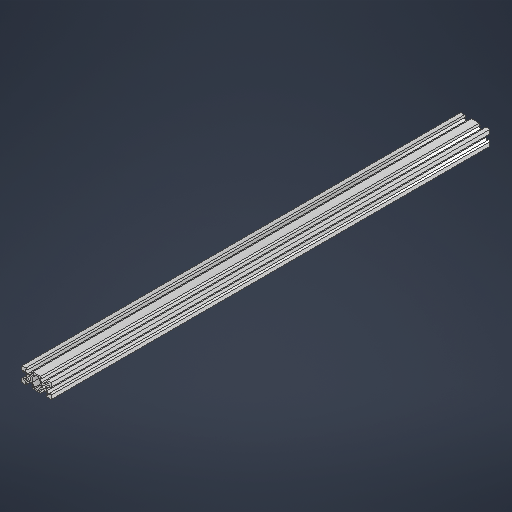
# Autodesk Inventor part: vslot_2040_100mm
Saved by Autodesk Inventor 2026 (Build 300175050, 175E)
## iProperties
Created: 2025-11-10
Part Number: vslot_2040_100mm
Material: Generic
Document SubType Name: Modeling
Designer: habbo
Density: 1 g/cm^3
Appearance: Aluminum - Polished
Author: habbo
Autodesk Inventor part; units mm, degrees
ref_plane "YZ Plane" through (0, 0, 0) normal (1, 0, 0) x (0, 1, 0)
ref_plane "XZ Plane" through (0, 0, 0) normal (0, 1, 0) x (-1, 0, 0)
ref_plane "XY Plane" through (0, 0, 0) normal (0, 0, 1) x (1, 0, 0)
sketch "Sketch1" plane through (0, 0, 0) normal (0, 0, 1) x (1, 0, 0)
  line L0 (4.5, 8.2) -> (4.5, 6.5562)
  line L1 (6.9, 8.2) -> (4.5, 8.2)
  line L2 (5.3896, 10) -> (6.9, 8.2)
  line L3 (-5.3896, 10) -> (5.3896, 10)
  line L4 (-5.3896, 10) -> (-6.9, 8.2)
  line L5 (-6.9, 8.2) -> (-4.5, 8.2)
  line L6 (-4.5, 8.2) -> (-4.5, 6.5562)
  line L7 (-4.5, 6.5562) -> (-7.1607, 3.9)
  line L8 (-9.4804, 3.8998) -> (-7.1607, 3.9)
  line L9 (-9.4804, 3.8998) -> (-10, 3.5998)
  line L10 (-10.5196, 3.8998) -> (-10, 3.5998)
  line L11 (-12.8393, 3.9) -> (-10.5196, 3.8998)
  line L12 (-15.5, 6.5562) -> (-12.8393, 3.9)
  line L13 (-15.5, 8.2) -> (-15.5, 6.5562)
  line L14 (-13.1, 8.2) -> (-15.5, 8.2)
  line L15 (-14.6104, 10) -> (-13.1, 8.2)
  line L16 (-20, 10) -> (-14.6104, 10)
  line L17 (-20, 10) -> (-20, 4.6104)
  line L18 (-20, 4.6104) -> (-18.2, 3.1)
  line L19 (-18.2, 3.1) -> (-18.2, 5.5)
  line L20 (-16.5562, 5.5) -> (-18.2, 5.5)
  line L21 (-16.5562, 5.5) -> (-13.9, 2.8393)
  line L22 (-13.9, 0.5196) -> (-13.9, 2.8393)
  line L23 (-13.9, 0.5196) -> (-13.6, 0)
  line L24 (-13.6, 0) -> (-13.9, -0.5196)
  line L25 (-13.9, -2.8393) -> (-13.9, -0.5196)
  line L26 (-16.5562, -5.5) -> (-13.9, -2.8393)
  line L27 (-16.5562, -5.5) -> (-18.2, -5.5)
  line L28 (-18.2, -3.1) -> (-18.2, -5.5)
  line L29 (-20, -4.6104) -> (-18.2, -3.1)
  line L30 (-20, -10) -> (-20, -4.6104)
  line L31 (-20, -10) -> (-14.6104, -10)
  line L32 (-14.6104, -10) -> (-13.1, -8.2)
  line L33 (-13.1, -8.2) -> (-15.5, -8.2)
  line L34 (-15.5, -8.2) -> (-15.5, -6.5562)
  line L35 (-15.5, -6.5562) -> (-12.8393, -3.9)
  line L36 (-12.8393, -3.9) -> (-10.5196, -3.9002)
  line L37 (-10.5196, -3.9002) -> (-10, -3.6002)
  line L38 (-9.4804, -3.9002) -> (-10, -3.6002)
  line L39 (-9.4804, -3.9002) -> (-7.1604, -3.9002)
  line L40 (-4.5, -6.5562) -> (-7.1604, -3.9002)
  line L41 (-4.5, -8.2) -> (-4.5, -6.5562)
  line L42 (-6.9, -8.2) -> (-4.5, -8.2)
  line L43 (-5.3896, -10) -> (-6.9, -8.2)
  line L44 (-5.3896, -10) -> (5.3896, -10)
  line L45 (5.3896, -10) -> (6.9, -8.2)
  line L46 (6.9, -8.2) -> (4.5, -8.2)
  line L47 (4.5, -8.2) -> (4.5, -6.5562)
  line L48 (4.5, -6.5562) -> (7.1607, -3.9)
  line L49 (9.4808, -3.9) -> (7.1607, -3.9)
  line L50 (9.4808, -3.9) -> (10, -3.6002)
  line L51 (10.5192, -3.9) -> (10, -3.6002)
  line L52 (12.8393, -3.9) -> (10.5192, -3.9)
  line L53 (15.5, -6.5562) -> (12.8393, -3.9)
  line L54 (15.5, -8.2) -> (15.5, -6.5562)
  line L55 (13.1, -8.2) -> (15.5, -8.2)
  line L56 (14.6104, -10) -> (13.1, -8.2)
  line L57 (20, -10) -> (14.6104, -10)
  line L58 (20, -10) -> (20, -4.6104)
  line L59 (20, -4.6104) -> (18.2, -3.1)
  line L60 (18.2, -3.1) -> (18.2, -5.5)
  line L61 (16.5562, -5.5) -> (18.2, -5.5)
  line L62 (16.5562, -5.5) -> (13.9, -2.8393)
  line L63 (13.9, -2.8393) -> (13.9, -0.5196)
  line L64 (13.6, 0) -> (13.9, -0.5196)
  line L65 (13.9, 0.5196) -> (13.6, 0)
  line L66 (13.9, 0.5196) -> (13.9, 2.8393)
  line L67 (16.5562, 5.5) -> (13.9, 2.8393)
  line L68 (16.5562, 5.5) -> (18.2, 5.5)
  line L69 (18.2, 3.1) -> (18.2, 5.5)
  line L70 (20, 4.6104) -> (18.2, 3.1)
  line L71 (20, 10) -> (20, 4.6104)
  line L72 (20, 10) -> (14.6104, 10)
  line L73 (14.6104, 10) -> (13.1, 8.2)
  line L74 (13.1, 8.2) -> (15.5, 8.2)
  line L75 (15.5, 8.2) -> (15.5, 6.5562)
  line L76 (15.5, 6.5562) -> (12.8481, 3.8998)
  line L77 (10.5196, 3.8998) -> (12.8481, 3.8998)
  line L78 (10.5196, 3.8998) -> (10, 3.5998)
  line L79 (9.4804, 3.8998) -> (10, 3.5998)
  line L80 (7.1519, 3.8998) -> (9.4804, 3.8998)
  line L81 (4.5, 6.5562) -> (7.1519, 3.8998)
  circle A0 centre (-10, 0) radius 2
  circle A1 centre (10, 0) radius 2
  line L82 (6.1, 2.8393) -> (2.3832, 6.5562)
  line L83 (6.1, 2.8393) -> (6.1, -2.8393)
  line L84 (6.1, -2.8393) -> (2.3769, -6.5562)
  line L85 (2.3769, -6.5562) -> (2.3769, -8.2)
  line L86 (-2.3769, -8.2) -> (2.3769, -8.2)
  line L87 (-2.3769, -6.5562) -> (-2.3769, -8.2)
  line L88 (-6.1, -2.8393) -> (-2.3769, -6.5562)
  line L89 (-6.1, 2.8393) -> (-6.1, -2.8393)
  line L90 (-6.1, 2.8393) -> (-2.3832, 6.5562)
  line L91 (-2.3832, 6.5562) -> (-2.3832, 8.2)
  line L92 (-2.3832, 8.2) -> (2.3832, 8.2)
  line L93 (2.3832, 6.5562) -> (2.3832, 8.2)
  point P0 (0, 0)
  point P1 (0, 0)
  constraints: 188 end point, 2 centre point
extrude "Extrusion1" add sketch "Sketch1" along normal mid plane 600
body "Solid1"
